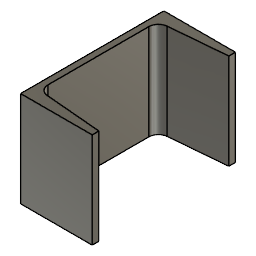
C-150×75×6.5×10 (Autodesk Fusion 360 design; units mm, degrees)
Autodesk Fusion 360 part; units mm, degrees
note: some values were not read from the file. Set by a fixed rule: which sketch regions a step uses.
sketch "スケッチ1" plane through (0, 0, 0) normal (0, 0, 1) x (1, 0, 0)
  line L0 (6.5, 127.8402) -> (6.5, 22.1598)
  line L1 (0, 150) -> (0, 0)
  line L2 (0, 0) -> (75, 0)
  line L3 (15.6284, 12.1979) -> (75, 7.0035)
  arc A0 (6.5, 22.1598) -> (15.6284, 12.1979) centre (16.5, 22.1598) ccw
  line L4 (75, 7.0035) -> (75, 0)
  line L5 (75, 142.9965) -> (15.6284, 137.8021)
  line L6 (0, 150) -> (75, 150)
  arc A1 (15.6284, 137.8021) -> (6.5, 127.8402) centre (16.5, 127.8402) ccw
  line L7 (75, 150) -> (75, 142.9965)
extrude "押し出し1" add sketch "スケッチ1" along normal blind 100
